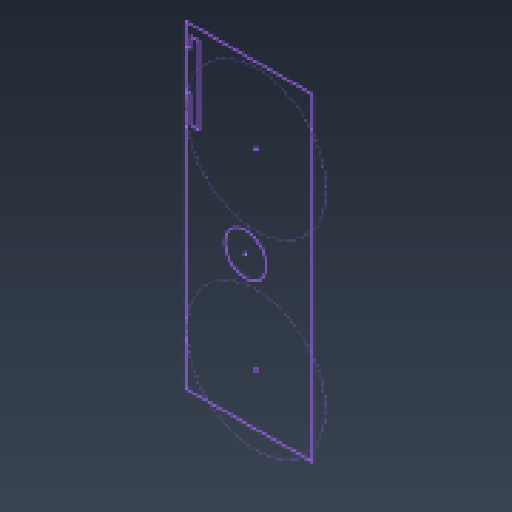
# Autodesk Inventor part: LeftGearboxCoverr
Saved by Autodesk Inventor 2026.2 (Build 302298010, 298A)
## iProperties
Created: 2026-04-13
Part Number: LeftGearboxCoverr
Material: Generic
Document SubType Name: Modeling
Designer: szymo
Density: 1 g/cm^3
Appearance: Default
Author: szymo
Autodesk Inventor part; units mm, degrees
ref_plane "YZ Plane" through (0, 0, 0) normal (1, 0, 0) x (0, 1, 0)
ref_plane "XZ Plane" through (0, 0, 0) normal (0, 1, 0) x (-1, 0, 0)
ref_plane "XY Plane" through (0, 0, 0) normal (0, 0, 1) x (1, 0, 0)
sketch "Sketch1" plane through (0, 0, 0) normal (0, 0, 1) x (1, 0, 0)
  circle A0 centre (14.7, -55.6371) radius 14.7 construction
  circle A1 centre (12.35, -35.2722) radius 5
  circle A2 centre (14.7, -14.7) radius 14.7 construction
  line L0 (27.4, -65.8371) -> (0, -65.8371)
  line L1 (0, -65.8371) -> (0, 0)
  line L2 (0, 0) -> (27.4, 0)
  line L3 (27.4, 0) -> (27.4, -65.8371)
  line L4 (2.5, -1) -> (2.5, -9.4261)
  line L5 (2.5, -1) -> (1, -1)
  line L6 (1, -1) -> (1, -3.5)
  line L7 (1, -3.5) -> (0, -3.5)
  line L8 (2.5, -9.4261) -> (2.5, -17.5)
  line L9 (2.5, -17.5) -> (1, -17.5)
  line L10 (1, -17.5) -> (1, -15)
  line L11 (1, -15) -> (0, -15)
  line L12 (7.8075, -4.272) -> (12.2251, -8.6896) construction
  arc A3 (12.2251, -8.6896) -> (8.6896, -12.2251) centre (14.7, -14.7) ccw construction
  line L13 (8.6896, -12.2251) -> (4.272, -7.8075) construction
  arc A4 (7.8075, -4.272) -> (4.272, -7.8075) centre (14.7, -14.7) ccw construction
  line L14 (7.8075, -4.272) -> (27.4, -4.272)
  line L15 (7.8075, -4.272) -> (2.5, -4.272)
  line L16 (2.5, -12.5) -> (27.4, -12.5)
  line L17 (0, -19.5) -> (27.4, -19.5)
  circle A5 centre (14.7, -55.6371) radius 4
  circle A6 centre (9.002, -47.4193) radius 1.25
  line L18 (23.1, -12.5) -> (23.1, -4.272)
  circle A7 centre (14.7, -55.6371) radius 14.7 projected
  circle A8 centre (14.7, -55.6371) radius 14 projected
  line L19 (18.8355, -20.9568) -> (21.7016, -23.8229) projected
  arc A9 (21.7016, -23.8229) -> (23.8229, -21.7016) centre (14.7, -14.7) ccw projected
  line L20 (23.8229, -21.7016) -> (20.9568, -18.8355) projected
  arc A10 (18.8355, -20.9568) -> (20.9568, -18.8355) centre (14.7, -14.7) ccw projected
  arc A11 (7.6984, -5.5771) -> (5.5771, -7.6984) centre (14.7, -14.7) ccw projected
  line L21 (5.5771, -7.6984) -> (8.4432, -10.5645) projected
  arc A12 (10.5645, -8.4432) -> (8.4432, -10.5645) centre (14.7, -14.7) ccw projected
  line L22 (10.5645, -8.4432) -> (7.6984, -5.5771) projected
  circle A13 centre (14.7, -14.7) radius 5 projected
  circle A14 centre (14.7, -14.7) radius 14 projected
  circle A15 centre (14.7, -14.7) radius 14.7 projected
  circle A16 centre (14.7, -14.7) radius 14 projected
  circle A17 centre (12.35, -35.2722) radius 5 projected
  circle A18 centre (12.35, -35.2722) radius 5.4 projected
  line L23 (1.5, -1) -> (1.5, -17) projected
  line L24 (2.5, -1) -> (1.5, -1) projected
  line L25 (2.5, -17) -> (2.5, -1) projected
  line L26 (2.5, -17) -> (1.5, -17) projected
  circle A19 centre (9.002, -47.4193) radius 1.25 projected
  arc A20 (10.0792, -44.7807) -> (10.0684, -43.3569) centre (6.4384, -44.0965) ccw projected
  arc A21 (10.4144, -44.9439) -> (10.0792, -44.7807) centre (9.002, -47.4193) ccw projected
  arc A22 (11.5418, -44.0742) -> (10.4144, -44.9439) centre (13.1986, -47.3876) ccw projected
  arc A23 (11.9567, -44.4343) -> (11.5418, -44.0742) centre (9.002, -47.4193) ccw projected
  arc A24 (11.2542, -45.6728) -> (11.9567, -44.4343) centre (8.4432, -43.2599) ccw projected
  arc A25 (11.4629, -45.9817) -> (11.2542, -45.6728) centre (9.002, -47.4193) ccw projected
  arc A26 (12.874, -45.7923) -> (11.4629, -45.9817) centre (12.6522, -49.4902) ccw projected
  arc A27 (13.0533, -46.3116) -> (12.874, -45.7923) centre (9.002, -47.4193) ccw projected
  arc A28 (11.8257, -47.0329) -> (13.0533, -46.3116) centre (10.5978, -43.5377) ccw projected
  arc A29 (11.8519, -47.4048) -> (11.8257, -47.0329) centre (9.002, -47.4193) ccw projected
  arc A30 (13.1688, -47.9463) -> (11.8519, -47.4048) centre (11.1277, -51.0378) ccw projected
  arc A31 (13.0643, -48.4857) -> (13.1688, -47.9463) centre (9.002, -47.4193) ccw projected
  arc A32 (11.6405, -48.4965) -> (13.0643, -48.4857) centre (12.3247, -44.8557) ccw projected
  arc A33 (11.4774, -48.8317) -> (11.6405, -48.4965) centre (9.002, -47.4193) ccw projected
  arc A34 (12.347, -49.9591) -> (11.4774, -48.8317) centre (9.0336, -51.6159) ccw projected
  arc A35 (11.9869, -50.374) -> (12.347, -49.9591) centre (9.002, -47.4193) ccw projected
  arc A36 (10.7484, -49.6715) -> (11.9869, -50.374) centre (13.1614, -46.8605) ccw projected
  arc A37 (10.4395, -49.8802) -> (10.7484, -49.6715) centre (9.002, -47.4193) ccw projected
  arc A38 (10.629, -51.2913) -> (10.4395, -49.8802) centre (6.9311, -51.0695) ccw projected
  arc A39 (10.1096, -51.4706) -> (10.629, -51.2913) centre (9.002, -47.4193) ccw projected
  arc A40 (9.3883, -50.2429) -> (10.1096, -51.4706) centre (12.8835, -49.0151) ccw projected
  arc A41 (9.0165, -50.2692) -> (9.3883, -50.2429) centre (9.002, -47.4193) ccw projected
  arc A42 (8.4749, -51.5861) -> (9.0165, -50.2692) centre (5.3834, -49.545) ccw projected
  arc A43 (7.9356, -51.4816) -> (8.4749, -51.5861) centre (9.002, -47.4193) ccw projected
  arc A44 (7.9247, -50.0578) -> (7.9356, -51.4816) centre (11.5656, -50.742) ccw projected
  arc A45 (7.5895, -49.8946) -> (7.9247, -50.0578) centre (9.002, -47.4193) ccw projected
  arc A46 (6.4622, -50.7643) -> (7.5895, -49.8946) centre (4.8053, -47.4509) ccw projected
  arc A47 (6.0473, -50.4042) -> (6.4622, -50.7643) centre (9.002, -47.4193) ccw projected
  arc A48 (6.7498, -49.1657) -> (6.0473, -50.4042) centre (9.5607, -51.5786) ccw projected
  arc A49 (6.5411, -48.8568) -> (6.7498, -49.1657) centre (9.002, -47.4193) ccw projected
  arc A50 (5.1299, -49.0462) -> (6.5411, -48.8568) centre (5.3518, -45.3483) ccw projected
  arc A51 (4.9507, -48.5269) -> (5.1299, -49.0462) centre (9.002, -47.4193) ccw projected
  arc A52 (6.1783, -47.8056) -> (4.9507, -48.5269) centre (7.4062, -51.3008) ccw projected
  arc A53 (6.152, -47.4338) -> (6.1783, -47.8056) centre (9.002, -47.4193) ccw projected
  arc A54 (4.8352, -46.8922) -> (6.152, -47.4338) centre (6.8763, -43.8007) ccw projected
  arc A55 (4.9396, -46.3529) -> (4.8352, -46.8922) centre (9.002, -47.4193) ccw projected
  arc A56 (6.3634, -46.342) -> (4.9396, -46.3529) centre (5.6792, -49.9828) ccw projected
  arc A57 (6.5266, -46.0068) -> (6.3634, -46.342) centre (9.002, -47.4193) ccw projected
  arc A58 (5.6569, -44.8794) -> (6.5266, -46.0068) centre (8.9703, -43.2226) ccw projected
  arc A59 (6.0171, -44.4646) -> (5.6569, -44.8794) centre (9.002, -47.4193) ccw projected
  arc A60 (7.2555, -45.1671) -> (6.0171, -44.4646) centre (4.8426, -47.978) ccw projected
  arc A61 (7.5644, -44.9584) -> (7.2555, -45.1671) centre (9.002, -47.4193) ccw projected
  arc A62 (7.375, -43.5472) -> (7.5644, -44.9584) centre (11.0729, -43.7691) ccw projected
  arc A63 (7.8943, -43.368) -> (7.375, -43.5472) centre (9.002, -47.4193) ccw projected
  arc A64 (8.6156, -44.5956) -> (7.8943, -43.368) centre (5.1205, -45.8234) ccw projected
  arc A65 (8.9875, -44.5693) -> (8.6156, -44.5956) centre (9.002, -47.4193) ccw projected
  arc A66 (9.529, -43.2525) -> (8.9875, -44.5693) centre (12.6205, -45.2935) ccw projected
  arc A67 (10.0684, -43.3569) -> (9.529, -43.2525) centre (9.002, -47.4193) ccw projected
  circle A68 centre (23.925, -15.5491) radius 0.75
  circle A69 centre (4.725, -15.5491) radius 0.75
  circle A70 centre (14.325, -3) radius 0.75
  point P0 (5.6819, -44.9285)
  point P1 (6.1842, -44.5249)
  point P2 (7.3688, -43.7101)
  point P3 (7.9148, -43.3912)
  dimension "d23" = 8
  dimension "d26" = 2.5
  dimension "d29" = 2
  dimension "d30" = 6.3
  dimension "d32" = 19.5
  dimension "d33" = 7
  dimension "d34" = 0.5
  dimension "d35" = 0.5
  dimension "d36" = 2.5
  dimension "d37" = 2.5
  dimension "d38" = 1
  dimension "d39" = 1
  dimension "d40" = 1
  dimension "d41" = 1
  dimension "d42" = 4.5
  constraints: 38 end point, 11 point on line, 10 centre point, 10 coincident, 8 perpendicular, 5 tangent, 4 horizontal, 4 parallel, 4 point on circle, 1 collinear, 1 vertical, 11 other
  measures "d23" diameter of A5
  measures "d26" diameter of A6
  measures "d29" distance edge to line of A2 L3
  measures "d30" distance edge to line of A2 L18
  measures "d32" distance between parallel lines of L17 L2
  measures "d33" distance between parallel lines of L17 L16
  measures "d34" distance between parallel lines of L9 L26
  measures "d35" distance between parallel lines of L10 L23
  measures "d36" distance between parallel lines of L11 L9
  measures "d37" distance between parallel lines of L7 L5
  measures "d38" distance between parallel lines of L12 L22
  measures "d39" distance between parallel lines of L13 L21
  measures "d40" radial gap between concentric circles of A12 A3
  measures "d41" radial gap between concentric circles of A11 A4
  measures "d42" distance edge to line of A0 L0
extrude "Extrusion3" add sketch "Sketch1" against normal blind 2 contours L0 A7 L3 | L0 A8 L3 A7 | L0 A8 A58 A57 A56 A55 A54 A53 A52 A51 A50 A49 A48 A47 A46 A45 A44 A43 A42 A41 A40 A39 A38 A37 A36 A35 A34 A33 A32 A31 A30 A29 A28 A27 A26 A25 A24 A23 A22 A21 A20 A67 A66 A65 A64 L3 | A7 L3 A8 A64 A63 A62 A60 A59 A58 L0 | L0 L1 A7 | L1 L17 A15 L3 A7 | A58 A59 A60 A8 | A8 A60 A61 A62 A64 A65 A66 A67 A20 A21 A22 A23 A24 A25 A26 A27 A28 A29 A30 A31 A32 A33 A34 A35 A36 A37 A38 A39 A40 A41 A42 A43 A44 A45 A46 A47 A48 A49 A50 A51 A52 A53 A54 A55 A56 A57 A58 | L1 L11 A15 L17 | A8 A62 A63 A64 | A15 L17 A14 L3 | A8 A62 A61 A60 | A15 L11 A14 L17 | A14 L17 A13 A10 L19 A9 L20 L3 | A14 L11 L10 L9 L8 L16 A13 L17 | L17 L20 A10 A13 L16 L3 | L1 L2 A15 L15 L4 L5 L6 L7 | A13 L16 L17 | L17 A13 | L20 A9 L19 A10 L17 | L17 A10 L20 | L14 A15 L2 L3 | L14 A14 L15 A15 | A15 L15 A14 L4 | L4 L15 A15 | A13 L16 | L16 L8 L4 A14 L15 L14 L18 A13 | L14 L15 A14 | A5 | A6 | L22 A12 L21 A11 | A18 | A68 | A69 | A70
ref_plane "Work Plane1" through (1, -19, -6.7) normal (0, 0, 1) x (1, 0, 0)
extrude "Extrusion4" add sketch "Sketch1" against normal up to surface (6.7 mm away) contours L1 L11 A15 L17 | A15 L11 A14 L17 | A14 L11 L10 L9 L8 L16 A13 L17 | L17 L20 A10 A13 L16 L3 | L1 L2 A15 L15 L4 L5 L6 L7 | A13 L16 L17 | L17 A10 L20 | L14 A15 L2 L3 | L14 A14 L15 A15 | A15 L15 A14 L4 | L4 L15 A15 | A13 L16 | L16 L8 L4 A14 L15 L14 L18 A13 | L14 L15 A14 | L22 A12 L21 A11 | A68 | A69 | A70
hole "Hole1" at (23.925, -15.5491, 0) at (4.725, -15.5491, 0) at (14.325, -3, 0) direction (0, 0, -1) diameter 3 end through all counterbore diameter 3.5 counterbore depth 0.5
extrude "Extrusion5" cut sketch "Sketch1" against normal blind 1.5 contours A5
extrude "Extrusion6" cut sketch "Sketch1" against normal blind 1.5 contours A6
body "Solid3"
